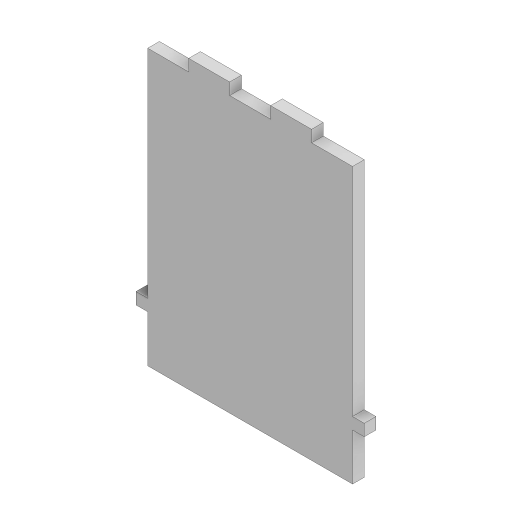
# Autodesk Inventor part: Bottom
Saved by Autodesk Inventor 2023.3 (Build 273359000, 359)
## iProperties
Created: 2024-06-25
Part Number: Bottom
Material: Generic
Document SubType Name: Modeling
Designer: David Zindović
Density: 1 g/cm^3
Appearance: Default
Author: David Zindović
Autodesk Inventor part; units mm, degrees
ref_plane "YZ Plane" through (0, 0, 0) normal (1, 0, 0) x (0, 1, 0)
ref_plane "XZ Plane" through (0, 0, 0) normal (0, 1, 0) x (-1, 0, 0)
ref_plane "XY Plane" through (0, 0, 0) normal (0, 0, 1) x (1, 0, 0)
sketch "Sketch1" plane through (0, 0, 0) normal (0, 0, 1) x (1, 0, 0)
  line L0 (-35, 47) -> (35, 47)
  line L1 (35, 47) -> (35, -47)
  line L2 (35, -47) -> (-35, -47)
  line L3 (-35, -47) -> (-35, 47)
  line L4 (-21, 47) -> (-7, 47)
  line L5 (-7, 47) -> (-7, 51)
  line L6 (-7, 51) -> (-21, 51)
  line L7 (-21, 51) -> (-21, 47)
  line L8 (7, 47) -> (21, 47)
  line L9 (21, 47) -> (21, 51)
  line L10 (21, 51) -> (7, 51)
  line L11 (7, 51) -> (7, 47)
  line L12 (-35, 9.4) -> (-35, 28.2)
  line L13 (-35, -31) -> (-39, -31)
  line L14 (-35, -47) -> (-35, -31)
  line L15 (0, 0) -> (0, 10.1242)
  line L16 (35, -31) -> (39, -31)
  line L17 (-35, -31) -> (-39, -31)
  line L18 (-39, -31) -> (-39, -27)
  line L19 (-39, -27) -> (-35, -27)
  line L20 (-35, -27) -> (-35, -31)
  line L21 (35, -31) -> (39, -31)
  line L22 (39, -31) -> (39, -27)
  line L23 (39, -27) -> (35, -27)
  line L24 (35, -27) -> (35, -31)
  point P0 (0, 47)
  point P1 (35, 0)
  point P2 (35, -31)
  point P3 (-37, -47)
  point P4 (-35, -27)
  point P5 (39, -31)
  point P6 (35, -27)
  dimension "d0" = 94
  dimension "d1" = 70
  dimension "d2" = 14
  dimension "d3" = 14
  dimension "d4" = 14
  dimension "d5" = 14
  dimension "d6" = 4
  dimension "d14" = 4
  dimension "d15" = 4
  dimension "d16" = 4
  dimension "d17" = 4
  dimension "d19" = 78
  constraints: 50 end point, 10 parallel, 6 horizontal, 5 perpendicular, 4 point on line, 3 horizontal alignment, 2 midpoint, 2 symmetric about line, 1 vertical, 1 vertical alignment
  measures "d0" distance of L0.end L1.end
  measures "d1" distance of L0.start L0.end
  measures "d2" distance of L5.end L6.end
  measures "d3" distance from line of L0.start L7
  measures "d4" distance of L9.end L10.end
  measures "d5" distance between parallel lines of L5 L11
  measures "d6" distance of L6.end L4.start
  measures "d14" distance of L18.end L19.end
  measures "d15" distance of L17.end L18.end
  measures "d16" distance of L23.end L22.end
  measures "d17" distance of L22.end L21.end
  measures "d19" distance from line of L18.end L6
extrude "Extrusion1" add sketch "Sketch1" along normal mid plane 4
equation "\"d2\" = 0.2 * d1"
equation "\"d3\" = d2"
equation "\"d4\" = d2"
equation "\"d5\" = d3"
body "Solid1"
